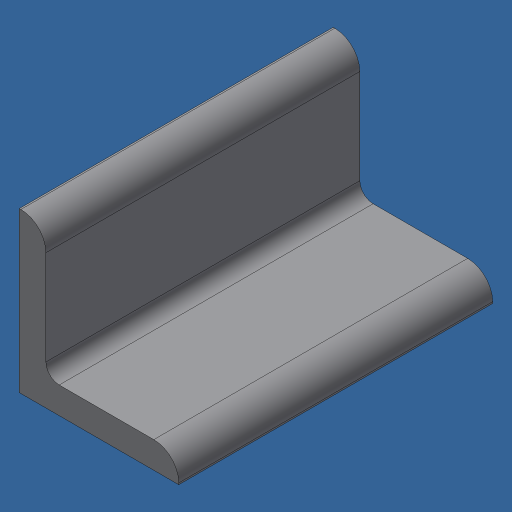
# Autodesk Inventor part: ANGLE IRON, 6 X 6 X 1 THK
Saved by Autodesk Inventor 2024.3 (Build 283343000, 343)
## iProperties
Category: _
Manager: _
Created: 2023-11-08
Part Number: ANGLE IRON, 6 X 6 X 1 THK
Checked By: 00
Engr Approved By: _
User Status: Work In Process
Material: Angle Iron
Description: ANGLE IRON, 6 X 6 X 1 THK
Document SubType Name: Modeling
Mfg Approved By: Stephen.Oerton
Designer: -
Mass: 16238.8 g
Surface Area: 1888.7 cm^2
Volume: 2066.01 cm^3
Density: 7.86 g/cm^3
Appearance: Grey (Light)
CN_MASS: 16.24
CN_SERVICEABLE: _
CL_runCount: 0
FIRST_DESCRIPTION: _
SECOND_DESCRIPTION: _
THIRD_DESCRIPTION: _
ModelCat: Uncategorized
ILogicPurgeVersion: 2.2.20.20
OnSaveVersion: 2.2.20.20
Subject: _
Author: -
Keywords: -
Revision Number: A
Autodesk Inventor part; units mm, degrees
ref_plane "YZ Plane" through (0, 0, 0) normal (1, 0, 0) x (0, 1, 0)
ref_plane "XZ Plane" through (0, 0, 0) normal (0, 1, 0) x (-1, 0, 0)
ref_plane "XY Plane" through (0, 0, 0) normal (0, 0, 1) x (1, 0, 0)
sketch "Sketch1" plane through (0, 0, 0) normal (0, 0, 1) x (1, 0, 0)
  line L0 (0, 0) -> (0, 152.4)
  line L1 (0, 152.4) -> (1.524, 152.4)
  line L2 (25.4, 128.524) -> (25.4, 38.1)
  line L3 (0, 0) -> (152.4, 0)
  line L4 (152.4, 0) -> (152.4, 1.524)
  line L5 (128.524, 25.4) -> (38.1, 25.4)
  arc A0 (25.4, 38.1) -> (38.1, 25.4) centre (38.1, 38.1) ccw
  arc A1 (25.4, 128.524) -> (1.524, 152.4) centre (1.524, 128.524) ccw
  arc A2 (152.4, 1.524) -> (128.524, 25.4) centre (128.524, 1.524) ccw
  line L6 (0, 188.8139) -> (0, -31.469) projected
  line L7 (-31.469, 0) -> (188.8139, 0) projected
  point P0 (0, 0)
  dimension "thickness" = 25.4
  dimension "d3" = 25.4
  dimension "LegSize" = 152.4
  dimension "d5" = 152.4
  dimension "radius" = 12.7
  dimension "d7" = 23.876
  dimension "d8" = 23.876
  dimension "d11" = 0
  dimension "d12" = 0
  constraints: 12 end point, 6 point on circle, 6 tangent, 4 parallel, 3 centre point, 1 perpendicular, 1 vertical
  measures "thickness" distance between parallel lines of L2 L0
  measures "d3" distance between parallel lines of L5 L3
  measures "LegSize" distance of L0.start L0.end
  measures "d5" distance of L0.start L3.end
  measures "radius" radius of A0
  measures "d7" radius of A1
  measures "d8" radius of A2
  measures "d11" distance between parallel lines of L3 L7
  measures "d12" distance between parallel lines of L0 L6
extrude "6\" X 6\" X 1\"" add sketch "Sketch1" along normal mid plane 300
equation "\"d3\" = thickness"
equation "\"d5\" = LegSize"
